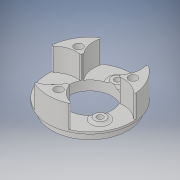
# Autodesk Inventor part: carrier_gear_hold_13.792
Saved by Autodesk Inventor 2019.4 (Build 234330000, 330)
## iProperties
Created: 2019-08-01
Part Number: carrier_gear_hold_13.792
Material: Generic
Document SubType Name: Modeling
Designer: cdi
Density: 1 g/cm^3
Appearance: Default
Author: cdi
Autodesk Inventor part; units mm, degrees
ref_plane "YZ Plane" through (0, 0, 0) normal (1, 0, 0) x (0, 1, 0)
ref_plane "XZ Plane" through (0, 0, 0) normal (0, 1, 0) x (-1, 0, 0)
ref_plane "XY Plane" through (0, 0, 0) normal (0, 0, 1) x (1, 0, 0)
sketch "Sketch1" plane through (0, 0, 0) normal (0, 1, 0) x (-1, 0, 0)
  circle A0 centre (0, 0) radius 22
  dimension "d0" = 44
  constraints: 1 centre point, 1 coincident
  measures "d0" diameter of A0
extrude "Extrusion1" add sketch "Sketch1" along normal blind 13
sketch "Sketch2" plane through (0, 0, 0) normal (0, -1, 0) x (1, 0, 0)
  circle A0 centre (0, 0) radius 19.96
  dimension "d3" = 39.92
  constraints: 1 centre point, 1 coincident
  measures "d3" diameter of A0
extrude "Extrusion2" add sketch "Sketch2" along normal blind 4
sketch "Sketch4" plane through (0, 13, 0) normal (0, 1, 0) x (1, 0, 0)
  circle A0 centre (0, 0) radius 14.344
  circle A1 centre (0, 14.344) radius 12.5
  dimension "d9" = 28.688
  dimension "d10" = 25
  constraints: 1 centre point, 1 coincident, 1 vertical alignment, 2 other
  measures "d10" diameter of A1
extrude "Extrusion4" cut sketch "Sketch4" against normal blind 12 contours A1 A0 | A0 A1 picked at (1.5859, 10.0886) picked at (-2.4785, 18.1439)
sketch "Sketch5" plane through (0, 1, 0) normal (0, 1, 0) x (1, 0, 0)
  circle A0 centre (0, 0) radius 14.344
  circle A1 centre (0, 14.344) radius 3
  dimension "d13" = 28.688
  dimension "d14" = 6
  constraints: 1 centre point, 1 coincident, 1 vertical alignment, 2 other
  measures "d14" diameter of A1
extrude "Extrusion5" add sketch "Sketch5" along normal blind 1 contours A1 A0 | A0 A1 picked at (0, 13.3207) picked at (0.0724, 15.3181)
sketch "Sketch6" plane through (0, 2, -14.344) normal (0, 1, 0) x (1, 0, 0)
  circle A0 centre (0, 0) radius 3 projected
  circle A1 centre (0, 0) radius 1.535
  point P0 (0, -14.344)
  dimension "d17" = 3.07
  constraints: 1 centre point, 1 coincident
  measures "d17" diameter of A1
extrude "Extrusion6" cut sketch "Sketch6" against normal blind 4.5 contours A1
pattern_circular "Circular Pattern1" count 3 over 360 about axis through (0, 0, 0) along (0, 1, 0) of "Extrusion4", "Extrusion5", "Extrusion6"
sketch "Sketch7" plane through (0, -4, 0) normal (0, -1, 0) x (1, 0, 0)
  circle A0 centre (0, 0) radius 11.5
  dimension "d23" = 23
  constraints: 1 centre point, 1 coincident
  measures "d23" diameter of A0
extrude "Extrusion7" cut sketch "Sketch7" against normal through all
fillet "Fillet1" radius 2 3 edges at (0, 1, -17.344) (-15.0203, 1, 8.672) (15.0203, 1, 8.672)
sketch "Sketch8" plane through (0, 13, 0) normal (0, 1, 0) x (1, 0, 0)
  circle A0 centre (0, -16.5) radius 1.5654
  point P0 (0, 0)
  dimension "d27" = 16.5
  constraints: 1 centre point
  measures "d27" distance of point (0, 0) A0.centre
hole "Hole1" at (0, 13, 16.5) direction (0, -1, 0) diameter 3.88 depth 10 countersink diameter 4.34 countersink angle 7
pattern_circular "Circular Pattern2" count 3 over 360 about axis through (0, 0, 0) along (0, 1, 0) of "Hole1"
fillet "Fillet2" radius 0.5 12 edges at (-9.5975, 7, -6.3354) (9.5975, 7, -6.3354) (10.2854, 7, -5.144) (0.6879, 7, 11.4794) (-11.7544, 7, -18.5966) (11.7544, 7, -18.5966) (21.9823, 7, -0.8813) (10.228, 7, 19.4779) (-10.2854, 7, -5.144) (-0.6879, 7, 11.4794) (-21.9823, 7, -0.8813) (-10.228, 7, 19.4779)
body "Solid1"
